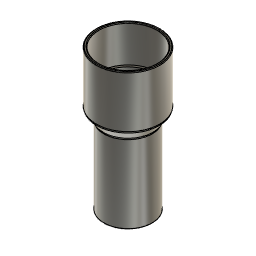
RHM8B-supporter (Autodesk Fusion 360 design; units mm, degrees)
Autodesk Fusion 360 part; units mm, degrees
sketch "スケッチ1" plane through (0, 0, 0) normal (0, 1, 0) x (1, 0, 0)
  line L0 (0, -73.6187) -> (0, 8) construction
  line L1 (-8.25, -0.25) -> (-8.25, -35)
  line L2 (-8.25, -35) -> (-10.2, -35)
  line L3 (-10.2, -35) -> (-10.2, -40)
  line L4 (-10.2, -40) -> (-11.1, -40)
  line L5 (-11.1, -40) -> (-11.1, -53.75)
  line L6 (-11.35, -54) -> (-11.85, -54)
  line L7 (-12.1, -53.75) -> (-12.1, -34.3198)
  line L8 (-11.9144, -33.7395) -> (-9.4356, -30.2605)
  line L9 (-9.25, -29.6802) -> (-9.25, -0.25)
  line L10 (-9, 0) -> (-8.5, 0)
  arc A0 (-9, 0) -> (-9.25, -0.25) centre (-9, -0.25) ccw
  arc A1 (-8.25, -0.25) -> (-8.5, 0) centre (-8.5, -0.25) ccw
  arc A2 (-9.4356, -30.2605) -> (-9.25, -29.6802) centre (-10.25, -29.6802) ccw
  arc A3 (-11.9144, -33.7395) -> (-12.1, -34.3198) centre (-11.1, -34.3198) ccw
  arc A4 (-12.1, -53.75) -> (-11.85, -54) centre (-11.85, -53.75) ccw
  arc A5 (-11.35, -54) -> (-11.1, -53.75) centre (-11.35, -53.75) ccw
  point P0 (-8.25, 0)
  point P1 (-11.0999, -54)
  point P2 (-12.1, -54)
  point P3 (-12.1, -34)
  point P4 (-9.25, -30)
  point P5 (-9.25, 0)
  dimension "d5" = 5
  dimension "d6" = 14
  dimension "d7" = 35
  dimension "d8" = 1
  dimension "d9" = 1
  dimension "d10" = 20
  dimension "d11" = 30
  dimension "d12" = 0.25
  dimension "d13" = 0.25
  dimension "d16" = 1
  dimension "d17" = 1
  dimension "d18" = 0.25
  dimension "d19" = 0.25
  dimension "d23" = 8.25
  dimension "d24" = 10.2
  dimension "d25" = 11.1
  constraint vertical L0
  constraint vertical L1
  constraint perpendicular L1 L2
  constraint perpendicular L2 L3
  constraint perpendicular L3 L4
  constraint perpendicular L4 L5
  constraint perpendicular L5 L6
  constraint perpendicular L6 L7
  constraint perpendicular L6 L9
  constraint perpendicular L1 L10
  constraint coincident origin L10
  constraint coincident P5 L9
  constraint coincident P5 L10
  constraint tangent L9 A0
  constraint tangent L10 A0
  constraint coincident P0 L1
  constraint coincident P0 L10
  constraint tangent L1 A1
  constraint tangent L10 A1
  constraint coincident P4 L9
  constraint coincident P4 L8
  constraint tangent L9 A2
  constraint tangent L8 A2
  constraint coincident P3 L7
  constraint coincident P3 L8
  constraint tangent L7 A3
  constraint tangent L8 A3
  constraint coincident P2 L6
  constraint coincident P2 L7
  constraint tangent L6 A4
  constraint tangent L7 A4
  constraint coincident P1 L6
  constraint tangent L6 A5
  constraint tangent L5 A5
  constraint coincident origin L0
  measures "d5" distance of L2.end L3.end
  measures "d6" distance of L4.end P1
  measures "d7" distance of P0 L1.end
  measures "d8" distance of L1 L9
  measures "d9" distance of L5 L7
  measures "d10" distance of P2 P3
  measures "d11" distance of P4 P5
  measures "d12" radius of A0
  measures "d13" radius of A1
  measures "d16" radius of A2
  measures "d17" radius of A3
  measures "d18" radius of A4
  measures "d19" radius of A5
  measures "d23" distance of L0 L1
  measures "d24" distance of L0 L3
  measures "d25" distance of L0 L5
revolve "回転6" add sketch "スケッチ1" angle 360 about axis through (0, 0, 73.6187) along (0, 0, -1)
revolve "回転4" [suppressed]
equation "d23 = ( 16.5 / 2 ) * 1 mm"
equation "d24 = ( 20.4 / 2 ) * 1 mm"
equation "d25 = ( 22.2 / 2 ) * 1 mm"
